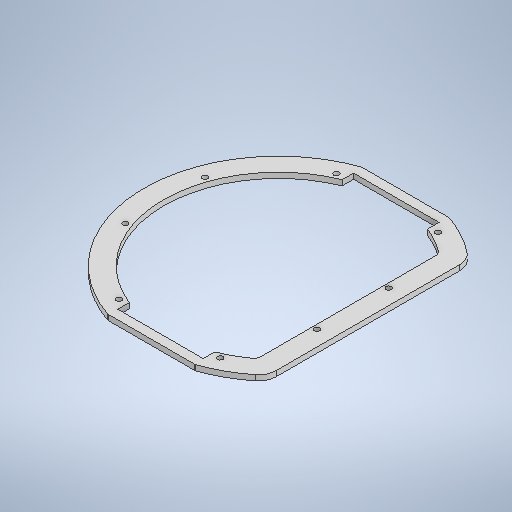
# Autodesk Inventor part: carcasa
Saved by Autodesk Inventor 2025.3 (Build 293356030, 356C)
## iProperties
Created: 2025-08-27
Part Number: carcasa
Material: Generic
Document SubType Name: Modeling
Designer: cdavi
Density: 1 g/cm^3
Appearance: Default
Author: cdavi
Autodesk Inventor part; units mm, degrees
ref_plane "YZ Plane" through (0, 0, 0) normal (1, 0, 0) x (0, 1, 0)
ref_plane "XZ Plane" through (0, 0, 0) normal (0, 1, 0) x (-1, 0, 0)
ref_plane "XY Plane" through (0, 0, 0) normal (0, 0, 1) x (1, 0, 0)
sketch "Sketch1" plane through (0, 0, 0) normal (0, 1, 0) x (-1, 0, 0)
  line L0 (23.1517, 65.9375) -> (-23.1517, 65.9375)
  line L1 (0, 0) -> (-50, 0) construction
  line L2 (24.013, 70.9375) -> (-24.013, 70.9375)
  line L3 (23.1517, -65.9375) -> (-23.5, -65.9375)
  line L4 (24.013, -70.9375) -> (-24.013, -70.9375)
  line L5 (0, 0) -> (0, 70.9375) construction
  line L6 (-45, 48.734) -> (-45, -48.734)
  line L7 (-50, 51.2348) -> (-50, -51.2348)
  arc A0 (-40.8333, -56.8563) -> (-23.5, -65.9375) centre (0, 0) ccw
  arc A1 (-46.1538, -59.117) -> (-24.6709, -70.8262) centre (0, 0) ccw
  arc A2 (24.6709, -70.8262) -> (24.6709, 70.8262) centre (0, 0) ccw
  arc A3 (-24.6709, 70.8262) -> (-46.1538, 59.117) centre (0, 0) ccw
  arc A4 (23.8326, -65.818) -> (23.8326, 65.818) centre (0, 0) ccw
  arc A5 (-23.8326, 65.818) -> (-40.8333, 56.8563) centre (0, 0) ccw
  arc A6 (-24.6709, -70.8262) -> (-24.013, -70.9375) centre (-24.013, -68.9375) ccw
  arc A7 (24.013, -70.9375) -> (24.6709, -70.8262) centre (24.013, -68.9375) ccw
  arc A8 (23.1517, -65.9375) -> (23.8326, -65.818) centre (23.1517, -63.9375) ccw
  arc A9 (23.8326, 65.818) -> (23.1517, 65.9375) centre (23.1517, 63.9375) ccw
  arc A10 (24.6709, 70.8262) -> (24.013, 70.9375) centre (24.013, 68.9375) ccw
  arc A11 (-23.1517, 65.9375) -> (-23.8326, 65.818) centre (-23.1517, 63.9375) ccw
  arc A12 (-24.013, 70.9375) -> (-24.6709, 70.8262) centre (-24.013, 68.9375) ccw
  arc A13 (-40.8333, 56.8563) -> (-45, 48.734) centre (-35, 48.734) ccw
  arc A14 (-46.1538, 59.117) -> (-50, 51.2348) centre (-40, 51.2348) ccw
  arc A15 (-50, -51.2348) -> (-46.1538, -59.117) centre (-40, -51.2348) ccw
  arc A16 (-45, -48.734) -> (-40.8333, -56.8563) centre (-35, -48.734) ccw
  point P0 (-24.349, 70.9375)
  point P1 (23.5, -65.9375)
  point P2 (24.349, -70.9375)
  point P3 (-24.349, -70.9375)
  point P4 (-50, -55.9017)
  point P5 (-45, 53.619)
  point P6 (-45, -53.619)
  point P7 (-50, 55.9017)
  point P8 (24.349, 70.9375)
  point P9 (23.5, 65.9375)
  point P10 (-23.5, 65.9375)
  dimension "d2" = 65.9375
  dimension "d4" = 5
  dimension "d6" = 45
  dimension "d7" = 5
  dimension "d8" = 2
  dimension "d9" = 10
  dimension "d10" = 70
  dimension "d11" = 75
  dimension "d12" = 70
  dimension "d13" = 75
  constraints: 45 point on circle, 22 tangent, 17 centre point, 16 end point, 11 point on line, 9 equal radius, 4 symmetric about line, 3 vertical, 2 coincident, 2 horizontal, 2 midpoint, 1 parallel
  measures "d2" distance between parallel lines of L1 L0
  measures "d4" distance between parallel lines of L0 L2
  measures "d6" distance between parallel lines of L6 L5
  measures "d7" distance between parallel lines of L7 L6
  measures "d8" radius of A6
  measures "d9" radius of A13
  measures "d10" radius of A4
  measures "d11" radius of A2
  measures "d12" radius of A0
  measures "d13" radius of A1
extrude "Extrusion1" add sketch "Sketch1" along normal blind 65
sketch "Sketch2" plane through (50, 0, 51.2348) normal (1, 0, 0) x (0, 0, -1)
  line L0 (51.2348, 0) -> (51.2348, 65) construction
  line L1 (99.9687, 65) -> (2.5008, 65) projected
  line L2 (-0.5914, 38) -> (19.4086, 38)
  line L3 (19.4086, 38) -> (19.4086, 26)
  line L4 (19.4086, 26) -> (-0.5914, 26)
  line L5 (-0.5914, 26) -> (-0.5914, 38)
  line L6 (0, 0) -> (102.4695, 0) projected
  line L7 (-19.5914, 0) -> (-19.5914, 65) projected
  line L8 (103.0609, 38) -> (83.0609, 38)
  line L9 (83.0609, 38) -> (83.0609, 26)
  line L10 (83.0609, 26) -> (103.0609, 26)
  line L11 (103.0609, 26) -> (103.0609, 38)
  dimension "d16" = 26
  dimension "d17" = 19
  dimension "d18" = 12
  dimension "d19" = 20
  constraints: 18 end point, 4 symmetric about line, 2 parallel, 1 horizontal, 1 midpoint, 1 perpendicular
  measures "d16" distance between parallel lines of L6 L4
  measures "d17" distance between parallel lines of L5 L7
  measures "d18" distance of L2.end L3.end
  measures "d19" distance of L2.start L2.end
extrude "Extrusion2" cut sketch "Sketch2" against normal blind 5
sketch "Sketch3" plane through (50, 0, 51.2348) normal (1, 0, 0) x (0, 0, -1)
  line L0 (3.568, 49.2223) -> (17.7975, 43.9952) construction
  line L1 (2.8909, 47.379) -> (17.1204, 42.1519)
  line L2 (18.4746, 45.8385) -> (4.2452, 51.0656)
  arc A0 (4.2452, 51.0656) -> (2.8909, 47.379) centre (3.568, 49.2223) ccw
  arc A1 (17.1204, 42.1519) -> (18.4746, 45.8385) centre (17.7975, 43.9952) ccw
  arc A2 (44.4296, 11.624) -> (34.6921, 2.9774) centre (43.8866, 2.4292) ccw construction
  arc A3 (44.531, 13.3402) -> (32.9759, 3.0797) centre (43.8866, 2.4292) ccw
  arc A4 (44.3283, 9.9077) -> (36.4083, 2.8751) centre (43.8866, 2.4292) ccw
  arc A5 (44.3283, 9.9077) -> (44.531, 13.3402) centre (44.4296, 11.624) ccw
  arc A6 (32.9759, 3.0797) -> (36.4083, 2.8751) centre (34.6921, 2.9774) ccw
  line L3 (51.2348, 0) -> (51.2348, 65) construction
  line L4 (99.5786, 47.379) -> (85.3491, 42.1519)
  line L5 (83.9949, 45.8385) -> (98.2243, 51.0656)
  arc A7 (99.5786, 47.379) -> (98.2243, 51.0656) centre (98.9015, 49.2223) ccw
  arc A8 (83.9949, 45.8385) -> (85.3491, 42.1519) centre (84.672, 43.9952) ccw
  point P0 (10.6828, 46.6088)
  constraints: 18 point on circle, 12 end point, 9 centre point, 8 tangent, 6 symmetric about line, 1 midpoint, 1 parallel, 2 other
extrude "Extrusion3" [suppressed]
extrude "Extrusion4" add sketch "Sketch1" along normal blind 3 from surface at 65 separate body contours A9 A4 A8 L3 A0 A16 L6 A13 A5 A11 L0 | A10 A2 A7 L4 A6 A1 A15 L7 A14 A3 A12 L2
sketch "Sketch5" plane through (-24.013, 68, 70.9375) normal (0, 1, 0) x (1, 0, 0)
  circle A0 centre (24.013, 70.9375) radius 8.5
  circle A1 centre (-5.987, 70.9375) radius 2.5
  line L0 (32.1371, 68.4375) -> (41.013, 68.4375)
  line L1 (41.013, 68.4375) -> (41.013, 73.4375)
  line L2 (41.013, 73.4375) -> (32.1371, 73.4375)
  point P0 (41.013, 70.9375)
  dimension "d26" = 17
  dimension "d27" = 5
  dimension "d31" = 5
  dimension "d32" = 17
  dimension "d47" = 30
  constraints: 6 end point, 2 centre point, 2 horizontal alignment, 2 perpendicular, 2 point on circle, 1 coincident, 1 horizontal, 1 midpoint
  measures "d26" diameter of A0
  measures "d27" diameter of A1
  measures "d31" distance between parallel lines of L2 L0
  measures "d32" distance from line of A0.centre L1
  measures "d47" distance of A0.centre A1.centre
extrude "Extrusion5" cut sketch "Sketch5" against normal through all bodies 2
sketch "Sketch6" plane through (0, 0, 0) normal (0, 1, 0) x (-1, 0, 0)
  circle A0 centre (0, 0) radius 67 construction
  arc A1 (-23.8326, 65.818) -> (-40.8333, 56.8563) centre (0, 0) ccw construction
  arc A2 (-40.8333, 56.8563) -> (-45, 48.734) centre (-35, 48.734) ccw construction
  line L0 (-45, -48.734) -> (-45, 48.734) construction
  arc A3 (-45, -48.734) -> (-40.8333, -56.8563) centre (-35, -48.734) ccw construction
  arc A4 (-40.8333, -56.8563) -> (-23.5, -65.9375) centre (0, 0) ccw construction
  line L1 (23.1517, -65.9375) -> (-23.5, -65.9375) construction
  arc A5 (23.8326, -65.818) -> (23.8326, 65.818) centre (0, 0) ccw construction
  line L2 (-23.1517, 65.9375) -> (23.1517, 65.9375) construction
  line L3 (24.013, 70.9375) -> (-24.013, 70.9375) projected
  arc A6 (-24.6709, 70.8262) -> (-46.1538, 59.117) centre (0, 0) ccw projected
  arc A7 (-46.1538, 59.117) -> (-50, 51.2348) centre (-40, 51.2348) ccw projected
  line L4 (-50, 51.2348) -> (-50, -51.2348) projected
  arc A8 (-50, -51.2348) -> (-46.1538, -59.117) centre (-40, -51.2348) ccw projected
  arc A9 (-46.1538, -59.117) -> (-24.6709, -70.8262) centre (0, 0) ccw projected
  line L5 (-24.013, -70.9375) -> (24.013, -70.9375) projected
  arc A10 (24.6709, -70.8262) -> (24.6709, 70.8262) centre (0, 0) ccw projected
  arc A11 (-22.7858, 59.8064) -> (-37.3333, 51.9829) centre (0, 0) ccw
  arc A12 (-37.3333, 51.9829) -> (-39, 48.734) centre (-35, 48.734) ccw
  line L6 (-39, 48.734) -> (-39, -48.734)
  arc A13 (-39, -48.734) -> (-37.3333, -51.9829) centre (-35, -48.734) ccw
  arc A14 (-37.3333, -51.9829) -> (-22.7858, -59.8064) centre (0, 0) ccw
  line L7 (-22.0737, -59.9375) -> (22.0737, -59.9375)
  line L8 (-22.0737, 59.9375) -> (22.0737, 59.9375)
  arc A15 (22.7858, -59.8064) -> (22.7858, 59.8064) centre (0, 0) ccw
  arc A16 (-8.124, -2.5) -> (-8.124, 2.5) centre (0, 0) ccw projected
  line L9 (0, 0) -> (63.1919, 22.2662) construction
  line L10 (0, 0) -> (75, 0) construction
  circle A17 centre (63.1919, 22.2662) radius 1.5
  line L11 (0, 0) -> (0, -67) construction
  circle A18 centre (28.3154, 60.7226) radius 1.5
  line L12 (28.3154, 60.7226) -> (0, 0) construction
  circle A19 centre (-41.5, 20) radius 1.5
  circle A20 centre (-28.3154, 60.7226) radius 1.5
  line L13 (-28.3154, 60.7226) -> (0, 0) construction
  arc A21 (-22.0737, 59.9375) -> (-22.7858, 59.8064) centre (-22.0737, 57.9375) ccw
  arc A22 (-22.7858, -59.8064) -> (-22.0737, -59.9375) centre (-22.0737, -57.9375) ccw
  arc A23 (22.0737, -59.9375) -> (22.7858, -59.8064) centre (22.0737, -57.9375) ccw
  arc A24 (22.7858, 59.8064) -> (22.0737, 59.9375) centre (22.0737, 57.9375) ccw
  arc A25 (-24.6709, -70.8262) -> (-24.013, -70.9375) centre (-24.013, -68.9375) ccw projected
  arc A26 (24.013, -70.9375) -> (24.6709, -70.8262) centre (24.013, -68.9375) ccw projected
  arc A27 (24.6709, 70.8262) -> (24.013, 70.9375) centre (24.013, 68.9375) ccw projected
  arc A28 (-24.013, 70.9375) -> (-24.6709, 70.8262) centre (-24.013, 68.9375) ccw projected
  circle A29 centre (63.1919, -22.2662) radius 1.5
  circle A30 centre (28.3154, -60.7226) radius 1.5
  circle A31 centre (-41.5, -20) radius 1.5
  circle A32 centre (-28.3154, -60.7226) radius 1.5
  line L14 (23.8326, 59.397) -> (23.8326, 65.818)
  line L15 (-23.8326, 59.397) -> (-23.8326, 65.818)
  line L16 (23.8326, 65.818) -> (-23.8326, 65.818)
  line L17 (23.8326, -59.397) -> (23.8326, -65.818)
  line L18 (-23.8326, -59.397) -> (-23.8326, -65.818)
  line L19 (23.8326, -65.818) -> (-23.8326, -65.818)
  point P0 (-22.4388, -59.9375)
  dimension "d33" = 134
  dimension "d34" = 6
  dimension "d35" = 6
  dimension "d36" = 6
  dimension "d37" = 19.41
  dimension "d38" = 25
  dimension "d39" = 3
  dimension "d40" = 20
  dimension "d41" = 3.5
  dimension "d42" = 25
  dimension "d44" = 2
  constraints: 28 end point, 25 point on circle, 18 centre point, 8 symmetric about line, 8 tangent, 6 equal radius, 2 coincident, 2 parallel, 1 perpendicular, 1 point on line, 1 vertical, 9 other
  measures "d33" diameter of A0
  measures "d34" radial gap between concentric circles of A1 A11
  measures "d35" distance between parallel lines of L2 L8
  measures "d36" radial gap between concentric circles of A5 A15
  measures "d37" angle of L10 L9
  measures "d38" angle of L11 L12
  measures "d39" diameter of A18
  measures "d40" distance from line of A19.centre L10
  measures "d41" distance from line of L0 A19.centre
  measures "d42" angle of L11 L13
  measures "d44" radius of A21
extrude "Extrusion6" add sketch "Sketch6" against normal blind 3 separate body
sketch "Sketch7" plane through (0, 0, 0) normal (0, 1, 0) x (1, 0, 0)
  line L0 (-23.8326, -69.0001) -> (-23.8326, 69.0001)
  line L1 (-23.8326, -59.397) -> (-23.8326, -65.818) projected
  line L2 (-73, 0) -> (-69.5603, 0)
  arc A0 (-24.6709, 70.8262) -> (-24.6709, -70.8262) centre (0, 0) ccw projected
  line L3 (-23.8326, 0) -> (-73, 0)
  arc A1 (-23.8326, 59.397) -> (-23.8326, -59.397) centre (0, 0) ccw
  arc A2 (-20.4784, 70.0688) -> (-20.4784, -70.0688) centre (0, 0) ccw
  line L4 (-73, 0) -> (-71.5, 0)
  line L5 (-71.5, 0) -> (-71.5, 8)
  line L6 (-71.5, 8) -> (-68.5, 8)
  line L7 (-68.5, 8) -> (-68.5, 0)
  line L8 (-71.5, 0) -> (-71.5, -8)
  line L9 (-71.5, -8) -> (-68.5, -8)
  line L10 (-68.5, -8) -> (-68.5, 0)
  line L11 (-69.4223, -17.1111) -> (-67.5078, -24.8786)
  line L12 (-67.5078, -24.8786) -> (-64.595, -24.1607)
  line L13 (-64.595, -24.1607) -> (-66.5095, -16.3931)
  line L14 (-68.424, -8.6256) -> (-66.5095, -16.3931)
  line L15 (-69.4223, -17.1111) -> (-71.3369, -9.3435)
  line L16 (-71.3369, -9.3435) -> (-68.424, -8.6256)
  line L17 (-63.3101, -33.2277) -> (-59.5923, -40.3114)
  line L18 (-59.5923, -40.3114) -> (-56.936, -38.9172)
  line L19 (-56.936, -38.9172) -> (-60.6537, -31.8335)
  line L20 (-64.3715, -24.7499) -> (-60.6537, -31.8335)
  line L21 (-63.3101, -33.2277) -> (-67.0279, -26.1441)
  line L22 (-67.0279, -26.1441) -> (-64.3715, -24.7499)
  line L23 (-53.5185, -47.4133) -> (-48.2135, -53.4014)
  line L24 (-48.2135, -53.4014) -> (-45.968, -51.412)
  line L25 (-45.968, -51.412) -> (-51.273, -45.4239)
  line L26 (-56.578, -39.4358) -> (-51.273, -45.4239)
  line L27 (-53.5185, -47.4133) -> (-58.8235, -41.4252)
  line L28 (-58.8235, -41.4252) -> (-56.578, -39.4358)
  line L29 (-40.6166, -58.8433) -> (-34.0328, -63.3879)
  line L30 (-34.0328, -63.3879) -> (-32.3286, -60.9189)
  line L31 (-32.3286, -60.9189) -> (-38.9124, -56.3744)
  line L32 (-45.4963, -51.8299) -> (-38.9124, -56.3744)
  line L33 (-40.6166, -58.8433) -> (-47.2005, -54.2988)
  line L34 (-47.2005, -54.2988) -> (-45.4963, -51.8299)
  line L35 (-25.3542, -66.8537) -> (-17.8741, -69.6905)
  line L36 (-17.8741, -69.6905) -> (-16.8103, -66.8855)
  line L37 (-16.8103, -66.8855) -> (-24.2904, -64.0486)
  line L38 (-31.7706, -61.2118) -> (-24.2904, -64.0486)
  line L39 (-25.3542, -66.8537) -> (-32.8344, -64.0168)
  line L40 (-32.8344, -64.0168) -> (-31.7706, -61.2118)
  line L41 (-8.6184, -70.9787) -> (-0.6767, -71.943)
  line L42 (-0.6767, -71.943) -> (-0.3151, -68.9649)
  line L43 (-0.3151, -68.9649) -> (-8.2568, -68.0006)
  line L44 (-16.1984, -67.0363) -> (-8.2568, -68.0006)
  line L45 (-8.6184, -70.9787) -> (-16.56, -70.0144)
  line L46 (-16.56, -70.0144) -> (-16.1984, -67.0363)
  line L47 (8.6184, -70.9787) -> (16.56, -70.0144)
  line L48 (16.56, -70.0144) -> (16.1984, -67.0363)
  line L49 (16.1984, -67.0363) -> (8.2568, -68.0006)
  line L50 (0.3151, -68.9649) -> (8.2568, -68.0006)
  line L51 (8.6184, -70.9787) -> (0.6767, -71.943)
  line L52 (0.6767, -71.943) -> (0.3151, -68.9649)
  line L53 (25.3542, -66.8537) -> (32.8344, -64.0168)
  line L54 (32.8344, -64.0168) -> (31.7706, -61.2118)
  line L55 (31.7706, -61.2118) -> (24.2904, -64.0486)
  line L56 (16.8103, -66.8855) -> (24.2904, -64.0486)
  line L57 (25.3542, -66.8537) -> (17.8741, -69.6905)
  line L58 (17.8741, -69.6905) -> (16.8103, -66.8855)
  line L59 (40.6166, -58.8433) -> (47.2005, -54.2988)
  line L60 (47.2005, -54.2988) -> (45.4963, -51.8299)
  line L61 (45.4963, -51.8299) -> (38.9124, -56.3744)
  line L62 (32.3286, -60.9189) -> (38.9124, -56.3744)
  line L63 (40.6166, -58.8433) -> (34.0328, -63.3879)
  line L64 (34.0328, -63.3879) -> (32.3286, -60.9189)
  line L65 (53.5185, -47.4133) -> (58.8235, -41.4252)
  line L66 (58.8235, -41.4252) -> (56.578, -39.4358)
  line L67 (56.578, -39.4358) -> (51.273, -45.4239)
  line L68 (45.968, -51.412) -> (51.273, -45.4239)
  line L69 (53.5185, -47.4133) -> (48.2135, -53.4014)
  line L70 (48.2135, -53.4014) -> (45.968, -51.412)
  line L71 (63.3101, -33.2277) -> (67.0279, -26.1441)
  line L72 (67.0279, -26.1441) -> (64.3715, -24.7499)
  line L73 (64.3715, -24.7499) -> (60.6537, -31.8335)
  line L74 (56.936, -38.9172) -> (60.6537, -31.8335)
  line L75 (63.3101, -33.2277) -> (59.5923, -40.3114)
  line L76 (59.5923, -40.3114) -> (56.936, -38.9172)
  line L77 (69.4223, -17.1111) -> (71.3369, -9.3435)
  line L78 (71.3369, -9.3435) -> (68.424, -8.6256)
  line L79 (68.424, -8.6256) -> (66.5095, -16.3931)
  line L80 (64.595, -24.1607) -> (66.5095, -16.3931)
  line L81 (69.4223, -17.1111) -> (67.5078, -24.8786)
  line L82 (67.5078, -24.8786) -> (64.595, -24.1607)
  line L83 (71.5, 0) -> (71.5, 8)
  line L84 (71.5, 8) -> (68.5, 8)
  line L85 (68.5, 8) -> (68.5, 0)
  line L86 (68.5, -8) -> (68.5, 0)
  line L87 (71.5, 0) -> (71.5, -8)
  line L88 (71.5, -8) -> (68.5, -8)
  line L89 (69.4223, 17.1111) -> (67.5078, 24.8786)
  line L90 (67.5078, 24.8786) -> (64.595, 24.1607)
  line L91 (64.595, 24.1607) -> (66.5095, 16.3931)
  line L92 (68.424, 8.6256) -> (66.5095, 16.3931)
  line L93 (69.4223, 17.1111) -> (71.3369, 9.3435)
  line L94 (71.3369, 9.3435) -> (68.424, 8.6256)
  line L95 (63.3101, 33.2277) -> (59.5923, 40.3114)
  line L96 (59.5923, 40.3114) -> (56.936, 38.9172)
  line L97 (56.936, 38.9172) -> (60.6537, 31.8335)
  line L98 (64.3715, 24.7499) -> (60.6537, 31.8335)
  line L99 (63.3101, 33.2277) -> (67.0279, 26.1441)
  line L100 (67.0279, 26.1441) -> (64.3715, 24.7499)
  line L101 (53.5185, 47.4133) -> (48.2135, 53.4014)
  line L102 (48.2135, 53.4014) -> (45.968, 51.412)
  line L103 (45.968, 51.412) -> (51.273, 45.4239)
  line L104 (56.578, 39.4358) -> (51.273, 45.4239)
  line L105 (53.5185, 47.4133) -> (58.8235, 41.4252)
  line L106 (58.8235, 41.4252) -> (56.578, 39.4358)
  line L107 (40.6166, 58.8433) -> (34.0328, 63.3879)
  line L108 (34.0328, 63.3879) -> (32.3286, 60.9189)
  line L109 (32.3286, 60.9189) -> (38.9124, 56.3744)
  line L110 (45.4963, 51.8299) -> (38.9124, 56.3744)
  line L111 (40.6166, 58.8433) -> (47.2005, 54.2988)
  line L112 (47.2005, 54.2988) -> (45.4963, 51.8299)
  line L113 (25.3542, 66.8537) -> (17.8741, 69.6905)
  line L114 (17.8741, 69.6905) -> (16.8103, 66.8855)
  line L115 (16.8103, 66.8855) -> (24.2904, 64.0486)
  line L116 (31.7706, 61.2118) -> (24.2904, 64.0486)
  line L117 (25.3542, 66.8537) -> (32.8344, 64.0168)
  line L118 (32.8344, 64.0168) -> (31.7706, 61.2118)
  line L119 (8.6184, 70.9787) -> (0.6767, 71.943)
  line L120 (0.6767, 71.943) -> (0.3151, 68.9649)
  line L121 (0.3151, 68.9649) -> (8.2568, 68.0006)
  line L122 (16.1984, 67.0363) -> (8.2568, 68.0006)
  line L123 (8.6184, 70.9787) -> (16.56, 70.0144)
  line L124 (16.56, 70.0144) -> (16.1984, 67.0363)
  line L125 (-8.6184, 70.9787) -> (-16.56, 70.0144)
  line L126 (-16.56, 70.0144) -> (-16.1984, 67.0363)
  line L127 (-16.1984, 67.0363) -> (-8.2568, 68.0006)
  line L128 (-0.3151, 68.9649) -> (-8.2568, 68.0006)
  line L129 (-8.6184, 70.9787) -> (-0.6767, 71.943)
  line L130 (-0.6767, 71.943) -> (-0.3151, 68.9649)
  line L131 (-25.3542, 66.8537) -> (-32.8344, 64.0168)
  line L132 (-32.8344, 64.0168) -> (-31.7706, 61.2118)
  line L133 (-31.7706, 61.2118) -> (-24.2904, 64.0486)
  line L134 (-16.8103, 66.8855) -> (-24.2904, 64.0486)
  line L135 (-25.3542, 66.8537) -> (-17.8741, 69.6905)
  line L136 (-17.8741, 69.6905) -> (-16.8103, 66.8855)
  line L137 (-40.6166, 58.8433) -> (-47.2005, 54.2988)
  line L138 (-47.2005, 54.2988) -> (-45.4963, 51.8299)
  line L139 (-45.4963, 51.8299) -> (-38.9124, 56.3744)
  line L140 (-32.3286, 60.9189) -> (-38.9124, 56.3744)
  line L141 (-40.6166, 58.8433) -> (-34.0328, 63.3879)
  line L142 (-34.0328, 63.3879) -> (-32.3286, 60.9189)
  line L143 (-53.5185, 47.4133) -> (-58.8235, 41.4252)
  line L144 (-58.8235, 41.4252) -> (-56.578, 39.4358)
  line L145 (-56.578, 39.4358) -> (-51.273, 45.4239)
  line L146 (-45.968, 51.412) -> (-51.273, 45.4239)
  line L147 (-53.5185, 47.4133) -> (-48.2135, 53.4014)
  line L148 (-48.2135, 53.4014) -> (-45.968, 51.412)
  line L149 (-63.3101, 33.2277) -> (-67.0279, 26.1441)
  line L150 (-67.0279, 26.1441) -> (-64.3715, 24.7499)
  line L151 (-64.3715, 24.7499) -> (-60.6537, 31.8335)
  line L152 (-56.936, 38.9172) -> (-60.6537, 31.8335)
  line L153 (-63.3101, 33.2277) -> (-59.5923, 40.3114)
  line L154 (-59.5923, 40.3114) -> (-56.936, 38.9172)
  line L155 (-69.4223, 17.1111) -> (-71.3369, 9.3435)
  line L156 (-71.3369, 9.3435) -> (-68.424, 8.6256)
  line L157 (-68.424, 8.6256) -> (-66.5095, 16.3931)
  line L158 (-64.595, 24.1607) -> (-66.5095, 16.3931)
  line L159 (-69.4223, 17.1111) -> (-67.5078, 24.8786)
  line L160 (-67.5078, 24.8786) -> (-64.595, 24.1607)
  dimension "d57" = 1.5
  dimension "d58" = 8
  dimension "d59" = 3
  dimension "d62" = 360
  constraints: 321 end point, 7 point on circle, 4 point on line, 2 centre point, 2 perpendicular, 2 symmetric about line, 1 coincident, 1 collinear, 1 horizontal, 1 midpoint, 314 other
  measures "d57" distance of L2.start L4.end
  measures "d58" distance of L4.end L5.end
  measures "d59" distance of L5.end L6.end
body "Solid1"
body "Solid2"
body "Solid3"
